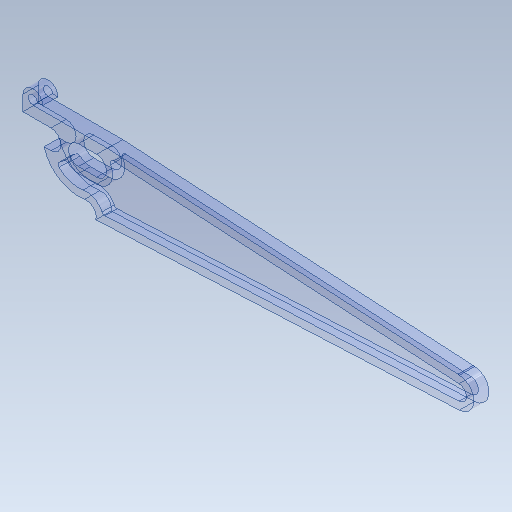
# Autodesk Inventor part: ウィング
Saved by Autodesk Inventor 2020.2 (Build 242310000, 310)
## iProperties
Created: 2020-04-12
Part Number: ウィング
Material: ポリカーボネート、クリア
Document SubType Name: Modeling
Designer: aoyama
Density: 1.2 g/cm^3
Appearance: トロピカル 青
Mass: 6.75592 g
Surface Area: 74.4038 cm^2
Volume: 5.62993 cm^3
Author: aoyama
Autodesk Inventor part; units mm, degrees
ref_plane "YZ Plane" through (0, 0, 0) normal (1, 0, 0) x (0, 1, 0)
ref_plane "XZ Plane" through (0, 0, 0) normal (0, 1, 0) x (-1, 0, 0)
ref_plane "XY Plane" through (0, 0, 0) normal (0, 0, 1) x (1, 0, 0)
sketch "スケッチ1" plane through (0, 0, 0) normal (0, 0, 1) x (1, 0, 0)
  line L0 (0, 0) -> (6, 0) construction
  line L1 (0, -3.25) -> (6, -3.25)
  line L2 (6, 3.25) -> (0, 3.25)
  arc A0 (0, 3.25) -> (0, -3.25) centre (0, 0) ccw
  arc A1 (6, -3.25) -> (6, 3.25) centre (6, 0) ccw
  line L3 (-15, 0) -> (-9, 0) construction
  line L4 (-9, 3.25) -> (-15, 3.25)
  arc A2 (-15, 3.25) -> (-18.25, 0) centre (-15, 0) ccw
  arc A3 (-9, -3.25) -> (-9, 3.25) centre (-9, 0) ccw
  line L5 (-9, 0) -> (0, 0)
  circle A4 centre (-15, 0) radius 3.25 construction
  circle A5 centre (2.604723, -14.772116) radius 3.25
  line L6 (0, 0) -> (2.604723, -14.772116) construction
  arc A6 (-11.29159, -3.25) -> (2.040366, -11.571491) centre (0, 0) ccw
  line L7 (0, 0) -> (125.4, 0)
  line L8 (125.340198, -9.986176) -> (5.767236, -15.521122)
  line L9 (-11.29159, -3.25) -> (-9, -3.25)
  arc A7 (-13.5, 8.25) -> (-15, 6.75) centre (-15, 8.25) ccw
  line L10 (-15, 8.25) -> (-15, 6.75) construction
  line L11 (-15, 3.25) -> (-18.25, 3.25)
  line L12 (-18.25, 3.25) -> (-18.25, 8.25)
  line L13 (-13.5, 8.25) -> (-11.75, 8.25)
  line L14 (-15, 6.75) -> (-9.617692, 6.75)
  arc A8 (-11.75, 0) -> (-11.29159, -3.25) centre (0, 0) ccw
  arc A9 (2.040366, -11.571491) -> (-11.75, 0) centre (0, 0) ccw construction
  line L15 (9.617692, 6.75) -> (125.4, 0)
  line L16 (-9.617692, 6.75) -> (9.617692, 6.75)
  line L17 (-15, 6.75) -> (-15, 0) construction
  arc A10 (-11.75, 8.25) -> (-18.25, 8.25) centre (-15, 8.25) ccw
  circle A11 centre (125.108999, -4.991525) radius 5
  point P0 (3, 0)
  point P1 (-12, 0)
  point P2 (2.040366, -11.571491)
  point P3 (124.817998, 0)
  dimension "d6" = 6.5
  dimension "d7" = 6.5
  dimension "d0" = 6.5
  dimension "d1" = 6
  dimension "d3" = 6.5
  dimension "d4" = 6
  dimension "d5" = 15
  dimension "d8" = 15
  dimension "d9" = 100
  dimension "d11" = 125.4
  dimension "d12" = 3
  dimension "d13" = 5
  dimension "d14" = 3.25
  dimension "d15" = 6.5
  dimension "d18" = 10
  constraints: 40 end point, 23 point on circle, 11 tangent, 10 centre point, 8 horizontal, 4 coincident, 2 midpoint, 2 parallel, 2 point on line, 2 vertical, 1 horizontal alignment, 6 other
  measures "d0" diameter of A1
  measures "d1" distance of L0.start L0.end
  measures "d3" diameter of A3
  measures "d4" distance of L3.start L3.end
  measures "d5" distance of L3.start point (0, 0)
  measures "d8" distance of L6.end point (0, 0)
  measures "d9" angle of L6 L5
  measures "d11" distance of L0.start L7.end
  measures "d12" diameter of A7
  measures "d13" distance from line of L10.start L4
  measures "d14" distance of L4.end L11.end
  measures "d15" diameter of A10
  measures "d18" diameter of A11
extrude "押し出し1" add sketch "スケッチ1" along normal blind 5 contours L1 A1 L7 A11 L8 A5 A6 L9 A3 L5 A0 | L5 A3 L4 L11 L12 A10 L13 A7 L14 L16 L15 A11 L7 A1 L2 A0 | L7 A11 picked at (123.673178, -4.767327)
sketch "スケッチ2" plane through (0, 0, 5) normal (0, 0, 1) x (1, 0, 0)
  arc A0 (-15, 6.75) -> (-13.5, 8.25) centre (-15, 8.25) ccw
  line L0 (-13.5, 8.25) -> (-11.75, 8.25)
  arc A1 (-11.75, 8.25) -> (-18.25, 8.25) centre (-15, 8.25) ccw
  line L1 (-18.25, 8.25) -> (-18.25, 3.25)
  arc A2 (-9, 3.25) -> (-9, -3.25) centre (-9, 0) ccw
  line L2 (-9, -3.25) -> (-11.29159, -3.25)
  arc A3 (-11.29159, -3.25) -> (2.040366, -11.571491) centre (0, 0) ccw
  arc A4 (2.040366, -11.571491) -> (5.767236, -15.521122) centre (2.604723, -14.772116) ccw
  line L3 (5.767236, -15.521122) -> (125.340198, -9.986176)
  arc A5 (125.340198, -9.986176) -> (125.4, 0) centre (125.108999, -4.991525) ccw
  line L4 (125.4, 0) -> (124.817998, 0)
  line L5 (124.817998, 0) -> (125.4, 0)
  line L6 (125.4, 0) -> (9.617692, 6.75)
  line L7 (0, 3.25) -> (6, 3.25)
  arc A6 (6, 3.25) -> (6, -3.25) centre (6, 0) ccw
  line L8 (6, -3.25) -> (0, -3.25)
  arc A7 (0, -3.25) -> (0, 3.25) centre (0, 0) ccw
  arc A8 (125.224598, -7.488851) -> (125.202485, -2.493273) centre (125.108999, -4.991525) ccw
  line L9 (125.224598, -7.488851) -> (8.045869, -12.912969)
  arc A9 (8.045869, -12.912969) -> (1.606246, -9.109472) centre (2.604723, -14.772116) ccw
  arc A10 (-7.416667, -5.527708) -> (1.606246, -9.109472) centre (0, 0) ccw
  arc A11 (-7.416667, -5.527708) -> (-9, 5.75) centre (-9, 0) ccw
  line L10 (125.254499, -2.495762) -> (9.041316, 4.279357)
  line L11 (6, 5.25) -> (0, 5.25)
  arc A12 (0, 5.25) -> (0, -5.25) centre (0, 0) ccw
  line L12 (0, -5.25) -> (6, -5.25)
  arc A13 (6, -5.25) -> (6, 5.25) centre (6, 0) ccw
  point P0 (-4.194444, -3.157394)
  point P1 (125.254499, -2.495762)
  point P2 (9.678702, 3.745617)
  point P3 (-4.194444, 3.157394)
  dimension "d19" = 2.5
  dimension "d20" = 2.5
  dimension "d21" = 2
  constraints: 14 centre point, 13 point on circle, 8 end point, 1 parallel, 7 other
  measures "d19" distance between parallel lines of L3 L9
  measures "d20" distance between parallel lines of L6 L10
  measures "d21" radial gap between concentric circles of A6 A13
extrude "押し出し2" cut sketch "スケッチ2" against normal blind 4 contours L9 A9 A10 A11 A12 L12 A13 L10 A8
fillet "フィレット1" radius 1.05 4 edges at (8.0459, -12.913, 3) (-7.4167, -5.5277, 3) (-4.1944, -3.1574, 3) (9.0413, 4.2794, 3)
